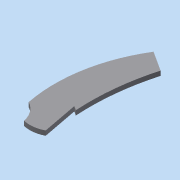
# Autodesk Inventor part: cueromango
Saved by Autodesk Inventor 2015 (Build 190159000, 159)
## iProperties
Created: 2017-10-06
Part Number: cueromango
Material: Generic
Document SubType Name: Modeling
Designer: macbook
Density: 1 g/cm^3
Appearance: Default
Author: macbook
Autodesk Inventor part; units mm, degrees
ref_plane "YZ Plane" through (0, 0, 0) normal (1, 0, 0) x (0, 1, 0)
ref_plane "XZ Plane" through (0, 0, 0) normal (0, 1, 0) x (-1, 0, 0)
ref_plane "XY Plane" through (0, 0, 0) normal (0, 0, 1) x (1, 0, 0)
sketch "Sketch1" plane through (0, 0, 0) normal (0, 0, 1) x (1, 0, 0)
  line L0 (-1.9526, -19.2383) -> (-0.4726, -26.9699)
  line L1 (-1.0107, -19.8473) -> (-1.9526, -19.2383)
  arc A0 (0.7413, -3.1056) -> (-1.0107, -19.8473) centre (49.2329, -16.6427) ccw
  line L2 (-3.5931, -0.3031) -> (0.7413, -3.1056)
  arc A1 (-3.5931, -0.3031) -> (-7.7014, -23.436) centre (23.9637, -17.1282) ccw
  arc A2 (-4.6851, -27.4777) -> (-7.7014, -23.436) centre (-10.5765, -28.728) ccw
  arc A3 (-4.6851, -27.4777) -> (-0.4726, -26.9699) centre (-3.2557, -21.6091) ccw
  constraints: 8 point on circle, 6 end point, 4 centre point
extrude "Extrusion1" add sketch "Sketch1" along normal blind 1
body "Solid1"
